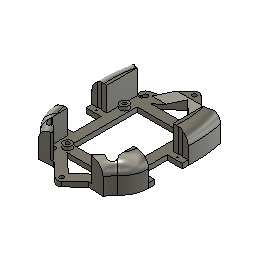
Arduino Base (Autodesk Fusion 360 design; units mm, degrees)
Autodesk Fusion 360 part; units mm, degrees
note: some values were not read from the file. Chosen so that the rebuilt part matches the saved one: which face or edge a step refers to; which pieces of a blend or face edit are solid. Set by a fixed rule: which sketch regions a step uses.
sketch "Arduino Base Sketch" plane through (0, 0, 0) normal (0, 1, 0) x (1, 0, 0)
  line L0 (27.5, -35) -> (-27.5, -35)
  line L1 (-27.5, -35) -> (-27.5, 35)
  line L2 (-27.5, 35) -> (27.5, 35)
  line L3 (27.5, 35) -> (27.5, -35)
  line L4 (27.5, -35) -> (-27.5, 35) construction
  line L5 (-27.5, -35) -> (27.5, 35) construction
  line L6 (0, 60) -> (0, -57) construction
  circle A0 centre (0, 55) radius 1.7
  circle A1 centre (0, 55) radius 4
  line L7 (27.5, 35) -> (2.7169, 57.9357)
  line L8 (-27.5, 35) -> (-2.7169, 57.9357)
  line L9 (-2.7163, 52.0638) -> (15.7218, 35)
  line L10 (-15.7218, 35) -> (2.7166, 52.064)
  line L11 (-21.0167, 41) -> (21.0167, 41)
  line L12 (-27.5, 10) -> (-40, 10)
  line L13 (-40, 10) -> (-40, 5.1)
  line L14 (-40, 5.1) -> (-27.5, 5.1)
  line L15 (-27.5, -17.9) -> (-40, -17.9)
  line L16 (-40, -17.9) -> (-40, -22.8)
  line L17 (-40, -22.8) -> (-27.5, -22.8)
  circle A2 centre (-33.75, 7.5) radius 0.5
  circle A3 centre (-33.75, -20.3) radius 0.5
  circle A4 centre (0, -55) radius 1.7
  circle A5 centre (0, -55) radius 4
  line L18 (2.7169, -57.9357) -> (27.5, -35)
  line L19 (-27.5, -35) -> (-2.7169, -57.9357)
  line L20 (-15.7218, -35) -> (2.7155, -52.063)
  line L21 (-2.7169, -52.0643) -> (15.7218, -35)
  line L22 (27.5, 10) -> (40, 10)
  line L23 (40, 10) -> (40, 5.1)
  line L24 (40, 5.1) -> (27.5, 5.1)
  line L25 (27.5, -17.9) -> (40, -17.9)
  line L26 (40, -17.9) -> (40, -22.8)
  line L27 (40, -22.8) -> (27.5, -22.8)
  circle A6 centre (33.75, 7.5) radius 0.5
  circle A7 centre (33.75, -20.3) radius 0.5
  line L28 (-19.5, -27) -> (-19.5, 27)
  line L29 (-19.5, 27) -> (19.5, 27)
  line L30 (19.5, 27) -> (19.5, -27)
  line L31 (19.5, -27) -> (-19.5, -27)
  line L32 (10.7515, 50.5) -> (-10.7515, 50.5)
  circle A8 centre (-19.13, -31.04) radius 1.5
  circle A9 centre (8.89, -31.04) radius 1.5
  circle A10 centre (-24.13, 21.2) radius 1.5
  circle A11 centre (24.13, 19.76) radius 1.5
  arc A12 (27.5, 35) -> (20.1607, 41.7922) centre (23.8303, 38.3961) ccw
  arc A13 (-20.1607, 41.7922) -> (-27.5, 35) centre (-23.8303, 38.3961) ccw
  arc A14 (21.6286, -40.4338) -> (27.5, -35) centre (24.5643, -37.7169) ccw
  arc A15 (-27.5, -35) -> (-21.6285, -40.4338) centre (-24.5643, -37.7169) ccw
  circle A16 centre (-24.5643, -37.7169) radius 2
  circle A17 centre (24.5643, -37.7169) radius 2
  circle A18 centre (23.8303, 38.3961) radius 2
  circle A19 centre (-23.8303, 38.3961) radius 2
  line L33 (0, 55) -> (0, 67) construction
  line L34 (0, 67) -> (-27, 67) construction
  line L35 (-40, 10) -> (-27, 67) construction
  line L36 (-33.5, 38.5) -> (-37.3999, 39.3894)
  arc A20 (-27, 67) -> (-40, 10) centre (68.6885, 15.1939) ccw
  line L37 (-10.7515, 50.5) -> (-34.2369, 50.5) construction
  arc A21 (-33.5, 38.5) -> (-27.5, 35) centre (-27.5, 41.8929) ccw
  line L38 (0, 67) -> (27, 67) construction
  line L39 (40, 10) -> (27, 67) construction
  line L40 (33.5, 38.5) -> (37.3999, 39.3894)
  arc A22 (27.5, 35) -> (33.5, 38.5) centre (27.5, 41.8929) ccw
  arc A23 (40, 10) -> (27, 67) centre (-68.6885, 15.1939) ccw
  arc A24 (-40, -22.8) -> (-25.5415, -41.5957) centre (-20.5538, -22.8) ccw construction
  arc A25 (25.603, -41.5797) -> (40, -22.8) centre (20.5533, -22.8) ccw construction
  line L41 (0, -55) -> (-25, -55)
  arc A26 (-40, -22.8) -> (-25, -55) centre (2.0613, -22.8) ccw construction
  arc A27 (-21.6285, -40.4338) -> (-20, -55) centre (-14.5193, -47.0131) ccw construction
  arc A28 (-40, -22.8) -> (-14.5193, -47.0131) centre (-15.7554, -22.8) ccw
  arc A29 (-25, -55) -> (-32.0323, -40.7684) centre (-46.551, -56.7958) ccw
  line L42 (-14.5193, -47.0131) -> (-26.9554, -47.648)
  circle A30 centre (-33.75, -20.3) radius 3
  circle A31 centre (-33.75, 7.5) radius 3
  circle A32 centre (33.75, 7.5) radius 3
  circle A33 centre (33.75, -20.3) radius 3
  line L43 (0, -55) -> (25, -55)
  arc A34 (20, -55) -> (21.6286, -40.4338) centre (14.5193, -47.0131) ccw construction
  arc A35 (14.5193, -47.0131) -> (40, -22.8) centre (15.7554, -22.8) ccw
  line L44 (27.5, -35) -> (32.0323, -40.7684)
  arc A36 (32.0323, -40.7684) -> (25, -55) centre (46.551, -56.7958) ccw
  line L45 (14.5193, -47.0131) -> (26.9554, -47.648)
  line L46 (-27.5, -35) -> (-32.0323, -40.7684)
  circle A37 centre (-24.13, 21.2) radius 3.5
  circle A38 centre (24.13, 19.76) radius 3.5
  circle A39 centre (8.89, -31.04) radius 3.5
  circle A40 centre (-19.13, -31.04) radius 3.5
  line L47 (-38.0384, 36.3961) -> (-23.8303, 36.3961)
  line L48 (-23.8303, 36.3961) -> (-23.8303, 35)
  line L49 (23.8303, 36.3961) -> (31.659, 36.3961)
  line L50 (23.8303, 36.3961) -> (23.8303, 35)
  circle A41 centre (-32.0323, -40.7684) radius 2 construction
  arc A42 (-35.0726, -37.4508) -> (-29.0297, -44.1201) centre (-32.0323, -40.7684) ccw construction
  line L51 (-33.5, 38.5) -> (-37.5988, 38.5)
  arc A43 (-24.8218, 43.2968) -> (-10.7515, 50.5) centre (-30.6228, 71.9718) ccw
  arc A44 (10.7515, 50.5) -> (24.8218, 43.2968) centre (30.6229, 71.9719) ccw
  dimension "d1" = 55
  dimension "d2" = 70
  dimension "d3" = 3.4
  dimension "d5" = 20
  dimension "d7" = 8
  dimension "d9" = 8
  dimension "d10" = 8
  dimension "d11" = 14
  dimension "d12" = 25
  dimension "d13" = 12.5
  dimension "d14" = 4.9
  dimension "d15" = 4.9
  dimension "d16" = 23
  dimension "d17" = 6.25
  dimension "d19" = 1
  dimension "d20" = 1
  dimension "d22" = 3.4
  dimension "d23" = 8
  dimension "d24" = 20
  dimension "d25" = 8
  dimension "d26" = 8
  dimension "d31" = 4.9
  dimension "d32" = 4.9
  dimension "d33" = 23
  dimension "d35" = 25
  dimension "d36" = 12.5
  dimension "d37" = 1
  dimension "d38" = 6.25
  dimension "d40" = 1
  dimension "d46" = 8
  dimension "d47" = 4.5
  dimension "d189" = 18.61
  dimension "d190" = 46.63
  dimension "d191" = 3
  dimension "d192" = 3
  dimension "d193" = 3
  dimension "d194" = 3
  dimension "d195" = 3.37
  dimension "d196" = 15.24
  dimension "d197" = 51.63
  dimension "d198" = 66.04
  dimension "d200" = 13.8
  dimension "d201" = 3.37
  dimension "d219" = 4
  dimension "d220" = 2
  dimension "d221" = 4
  dimension "d222" = 2
  dimension "d223" = 4
  dimension "d225" = 3
  dimension "d226" = 4
  dimension "d227" = 3
  dimension "d447" = 4
  dimension "d448" = 27
  dimension "d449" = 12
  dimension "d451" = 27
  dimension "d452" = 4
  dimension "d453" = 25
  dimension "d455" = 5
  dimension "d468" = 6
  dimension "d469" = 6
  dimension "d470" = 6
  dimension "d471" = 6
  dimension "d473" = 25
  dimension "d474" = 5
  dimension "d480" = 2.4
  dimension "d481" = 2.4
  dimension "d569" = 2
  dimension "d570" = 2
  dimension "d571" = 2
  dimension "d572" = 2
  dimension "d588" = 4
  dimension "d589" = 2.5
  constraint horizontal L0
  constraint perpendicular L0 L1
  constraint parallel L0 L2
  constraint parallel L1 L3
  constraint coincident L4 origin
  constraint coincident L5 origin
  constraint perpendicular L0 L6
  constraint coincident L6 A0.centre
  constraint concentric A0 A1
  constraint coincident A1 L7.end
  constraint coincident A1 L8.end
  constraint tangent A1 L7
  constraint tangent A1 L8
  constraint coincident A1 L9.start
  constraint coincident L2 L9.end
  constraint parallel L7 L9
  constraint coincident L2 L10.start
  constraint coincident A1 L10.end
  constraint parallel L8 L10
  constraint perpendicular L6 L11
  constraint coincident L7 L11.end
  constraint coincident L8 L11.start
  constraint coincident L1 L12.start
  constraint perpendicular L1 L12
  constraint perpendicular L12 L13
  constraint coincident L1 L14.end
  constraint perpendicular L1 L14
  constraint coincident L1 L15.start
  constraint perpendicular L1 L15
  constraint coincident L1 L17.end
  constraint perpendicular L1 L17
  constraint perpendicular L16 L17
  constraint collinear L13 L16
  constraint vertical A2.centre A3.centre
  constraint coincident L6 A4.centre
  constraint concentric A4 A5
  constraint coincident A5 L18.start
  constraint coincident A5 L19.end
  constraint tangent A5 L19
  constraint tangent A5 L18
  constraint coincident L0 L20.start
  constraint coincident A5 L20.end
  constraint coincident A5 L21.start
  constraint coincident L0 L21.end
  constraint parallel L19 L20
  constraint parallel L18 L21
  constraint coincident L3 L22.start
  constraint perpendicular L3 L22
  constraint coincident L3 L24.end
  constraint perpendicular L3 L24
  constraint coincident L3 L25.start
  constraint perpendicular L3 L25
  constraint perpendicular L24 L26
  constraint coincident L3 L27.end
  constraint perpendicular L3 L27
  constraint perpendicular L22 L23
  constraint collinear L23 L26
  constraint vertical A6.centre A7.centre
  constraint horizontal L32
  constraint coincident L8 L32.end
  constraint coincident L7 L32.start
  constraint coincident origin L6
  constraint horizontal A8.centre A9.centre
  constraint coincident L7 A12.centre
  constraint coincident L7 A12.end
  constraint coincident L8 A13.centre
  constraint coincident L8 A13.start
  constraint coincident L18 A14.centre
  constraint coincident L18 A14.start
  constraint coincident L19 A15.centre
  constraint coincident L19 A15.end
  constraint concentric A15 A16
  constraint concentric A14 A17
  constraint concentric A12 A18
  constraint concentric A13 A19
  constraint coincident A0.centre A1.centre
  constraint parallel L6 L33
  constraint perpendicular L6 L34
  constraint midpoint L35 L36.start
  constraint perpendicular L35 L36
  constraint coincident L36.end A20
  constraint parallel L32 L37
  constraint coincident A20 L37.end
  constraint perpendicular L33 L38
  constraint midpoint L39 L40.start
  constraint perpendicular L39 L40
  constraint coincident L40.end A23
  constraint tangent L2 A22
  constraint coincident A15 A24.end
  constraint tangent L16 A24
  constraint coincident A14 A25.start
  constraint tangent L26 A25
  constraint tangent A14 A25
  constraint coincident A4.centre A5.centre
  constraint perpendicular L6 L41
  constraint tangent L16 A26
  constraint tangent A15 A27
  constraint coincident L41 A27.end
  constraint coincident A27.centre A28.end
  constraint tangent L16 A28
  constraint parallel L5 L46
  constraint tangent A28 A29
  constraint coincident A28 A29.end
  constraint coincident A29 L42.end
  constraint tangent A28 L42
  constraint concentric A3 A30
  constraint concentric A2 A31
  constraint concentric A6 A32
  constraint concentric A7 A33
  constraint perpendicular L6 L43
  constraint coincident L43 A34.start
  constraint tangent A14 A34
  constraint tangent A25 A35
  constraint coincident A34.centre A35.start
  constraint parallel L4 L44
  constraint tangent A35 A36
  constraint coincident A35 L44.end
  constraint coincident A36 L45.end
  constraint tangent A35 L45
  constraint horizontal A3.centre A7.centre
  constraint horizontal A2.centre A6.centre
  constraint coincident A19 L47.end
  constraint horizontal L47
  constraint tangent A19 L47
  constraint coincident L2 L48.end
  constraint perpendicular L2 L48
  constraint coincident A18 L49.start
  constraint coincident A22 L49.end
  constraint tangent A18 L49
  constraint horizontal L49
  constraint coincident L2 L50.end
  constraint perpendicular L2 L50
  constraint coincident A29.end L46.end
  constraint coincident A28 A42.start
  constraint coincident A29 A42.end
  constraint coincident A20 L47.start
  constraint tangent L2 A21
  constraint coincident A20 L51.end
  constraint horizontal L51
  constraint tangent L8 A43
  constraint coincident A13 A43.start
  constraint tangent A13 A43
  constraint tangent L7 A44
  constraint coincident A12 A44.end
  constraint tangent A12 A44
  measures "d1" distance of L1.end L2.end
  measures "d2" distance of L0.end L1.end
  measures "d3" diameter of A0
  measures "d5" distance of L2 A0.centre
  measures "d7" diameter of A1
  measures "d9" distance of L7 L9
  measures "d10" distance of L8 L10
  measures "d11" distance of A0.centre L11
  measures "d12" distance of L2 L12
  measures "d13" distance of L1 L13
  measures "d14" distance of L12 L14
  measures "d15" distance of L15 L17
  measures "d16" distance of L14 L15
  measures "d17" distance of L1 A2.centre
  measures "d19" diameter of A2
  measures "d20" diameter of A3
  measures "d22" diameter of A4
  measures "d23" diameter of A5
  measures "d24" distance of L0 A4.centre
  measures "d25" distance of L19 L20
  measures "d26" distance of L18 L21
  measures "d31" distance of L25 L27
  measures "d32" distance of L22 L24
  measures "d33" distance of L24 L25
  measures "d35" distance of L2 L22
  measures "d36" distance of L3 L23
  measures "d37" diameter of A6
  measures "d38" distance of L3 A6.centre
  measures "d40" diameter of A7
  measures "d47" distance of A0.centre L32
  measures "d189" distance of L3 A9.centre
  measures "d190" distance of L3 A8.centre
  measures "d191" diameter of A8
  measures "d192" diameter of A9
  measures "d193" diameter of A10
  measures "d194" diameter of A11
  measures "d195" distance of L3 A11.centre
  measures "d196" distance of L2 A11.centre
  measures "d197" distance of L3 A10.centre
  measures "d198" distance of L2 A9.centre
  measures "d200" distance of L2 A10.centre
  measures "d201" distance of L1 A10.centre
  measures "d219" diameter of A16
  measures "d220" distance of A15 A16
  measures "d221" diameter of A17
  measures "d222" distance of A14 A17
  measures "d223" diameter of A18
  measures "d225" distance of A12 A18
  measures "d226" diameter of A19
  measures "d227" distance of A13 A19
  measures "d447" distance of L36.start L36.end
  measures "d448" distance of L33 L34.end
  measures "d449" distance of A0.centre L34
  measures "d451" distance of L33.end L38.end
  measures "d452" distance of L40.start L40.end
  measures "d453" distance of A4.centre L41.end
  measures "d455" distance of L41.end A27.end
  measures "d468" diameter of A30
  measures "d469" diameter of A31
  measures "d470" diameter of A32
  measures "d471" diameter of A33
  measures "d473" distance of A4.centre L43.end
  measures "d474" distance of L43.end A34.start
  measures "d480" distance of L14 A2.centre
  measures "d481" distance of L15 A3.centre
  measures "d588" diameter of A41
  measures "d589" distance of A41 A42
extrude "Extrude1" add sketch "Arduino Base Sketch" against normal blind 4 contours L0 A5 L18 L20 L21 A17 L43 | L0 L1 L2 L3 A37 A38 | L18 A14 A17 L44 | L3 L27 A14 A33 A35 L44 | A14 L44 | L3 L25 L27 A33 | L18 A14 A35 L44 | L0 A5 L19 L20 L21 A16 L41 | A5 L20 L21 | L25 L27 A33 | A35 A36 L45 | L1 L17 A15 A28 A30 L46 | A15 L46 | L19 A15 A16 L46 | A4 A5 L41 L43 | L3 L22 L24 A32 | L25 L26 L27 A33 | L1 L15 L17 A30 | L19 A15 A28 L46 | A5 L18 L43 | A4 A5 L41 L43 | A5 L19 L41 | L3 L22 L40 A22 A23 A32 A38 | L22 L24 A32 | L17 A30 | L15 L17 A30 | A28 A29 L42 | L3 A38 | L3 A38 | L22 A32 | L22 L23 L24 A32 | L1 L12 L14 A31 | L15 L16 L17 A30 | L1 L12 A20 A21 A31 A37 L47 | L12 L14 A31 | L1 A37 | L1 A37 | L12 A31 | L12 L13 L14 A31 | L2 L7 L9 L11 A18 L50 | L7 A12 A18 L49 | L7 A12 A44 | L2 L8 L10 L11 A19 L48 | L7 L9 L10 L11 L32 | L8 A13 A19 L47 | A20 A21 L47 L51 | L8 L9 L10 L11 L32 | L9 L10 L32 | L8 A13 A43 | L36 A20 L51 | A39 | A40
extrude "Extrude2" add sketch "Arduino Base Sketch" along normal blind 4 contours L7 L9 L10 L11 L32 | A1 L7 L10 L32 | L8 L9 L10 L11 L32 | L9 L10 L32 | A1 | A1 L9 L10 L32 | A1 L8 L9 L32
chamfer "Chamfer1" distance 10 distance2 4 2 edges at (15.1276, 4, -41) (-15.1276, 4, -41) measured on face at (10.9907, 4, -46.6452) measured on face at (10.9907, 4, -46.6452)
extrude "Extrude3" add sketch "Arduino Base Sketch" along normal blind 20 contours L3 L27 A14 A33 A35 L44 | L18 A14 A35 L44 | A35 A36 L45 | L1 L17 A15 A28 A30 L46 | A15 L46 | L19 A15 A28 L46 | L3 L22 L40 A22 A23 A32 A38 | A28 A29 L42 | L3 A38 | L1 L12 A20 A21 A31 A37 L47 | L1 A37 | A20 A21 L47 L51 | L36 A20 L51 picked at (27.524, 19.5485) picked at (-27.5324, 21.359)
fillet "Fillet1" radius 10 6 edges at (-39.7007, 20, -24.7833) (-37.9187, 20, 32.6279) (-29.1505, 20, 43.9548) (39.7007, 20, -24.7833) (37.9188, 20, 32.6279) (29.1505, 20, 43.9548)
extrude "Extrude5" add sketch "Arduino Base Sketch" along normal blind 3 contours L3 A38 | L1 A37 | A39 | A40 picked at (26.8767, 19.76) picked at (-26.8767, 21.2)
fillet "Fillet2" radius 1 4 edges at (14.5193, 10, 47.0131) (21.6286, 10, 40.4338) (-14.5193, 10, 47.0131) (-21.6285, 10, 40.4338)
equation "d3 = hingeBoltDia + 0.4 mm"
equation "d7 = strutsWidth"
equation "d9 = strutsWidth"
equation "d10 = strutsWidth"
equation "d11 = 10 mm + d7 / 2"
equation "d17 = d13 / 2"
equation "d19 = servoScrewHoles"
equation "d20 = servoScrewHoles"
equation "d22 = hingeBoltDia + 0.4 mm"
equation "d23 = strutsWidth"
equation "d25 = strutsWidth"
equation "d26 = strutsWidth"
equation "d37 = servoScrewHoles"
equation "d38 = d36 / 2"
equation "d40 = servoScrewHoles"
equation "d42 = -frameThickness"
equation "d46 = strutsWidth"
equation "d47 = 0.5 mm + d7 / 2"
equation "d48 = frameThickness"
equation "d189 = 17.78 mm + arduinoOffset"
equation "d190 = 45.8 mm + arduinoOffset"
equation "d195 = 2.54 mm + arduinoOffset"
equation "d197 = 50.8 mm + arduinoOffset"
equation "d451 = d448"
equation "d473 = d453"
equation "d474 = d455"
equation "hingeBoltDia = 3 mm"
equation "strutsWidth = 8 mm"
equation "frameThickness = 4 mm"
equation "arduinoOffset = 0.83 mm"
equation "servoScrewHoles = 1 mm"
named bodies: "Arduino Base"
